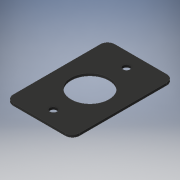
# Autodesk Inventor part: borracha isolamento prensa cabo
Saved by Autodesk Inventor 2019.4 (Build 234330000, 330)
## iProperties
Created: 2021-02-09
Part Number: borracha isolamento prensa cabo
Material: Borracha
Document SubType Name: Modeling
Designer: Lattes
Density: 0.93 g/cm^3
Appearance: Borracha - Preta
Author: Lattes
Autodesk Inventor part; units mm, degrees
ref_plane "YZ Plane" through (0, 0, 0) normal (1, 0, 0) x (0, 1, 0)
ref_plane "XZ Plane" through (0, 0, 0) normal (0, 1, 0) x (-1, 0, 0)
ref_plane "XY Plane" through (0, 0, 0) normal (0, 0, 1) x (1, 0, 0)
sketch "Esboço1" plane through (0, 0, 0) normal (0, 1, 0) x (-1, 0, 0)
  circle A0 centre (0, -15.425) radius 1.5
  circle A1 centre (0, 15.425) radius 1.5
  circle A2 centre (0, 0) radius 8
  line L0 (-14, 21.425) -> (14, 21.425)
  line L1 (14, 21.425) -> (14, -21.425)
  line L2 (14, -21.425) -> (-14, -21.425)
  line L3 (-14, -21.425) -> (-14, 21.425)
  dimension "d0" = 3
  dimension "d1" = 3
  dimension "d2" = 16
  constraints: 8 end point, 3 centre point, 2 parallel, 1 coincident, 1 horizontal, 1 perpendicular
  measures "d0" diameter of A0
  measures "d1" diameter of A1
  measures "d2" diameter of A2
extrude "Extrusão1" add sketch "Esboço1" along normal blind 1
fillet "Arredondamento1" radius 3 4 edges at (14, 0.5, 21.425) (-14, 0.5, 21.425) (14, 0.5, -21.425) (-14, 0.5, -21.425)
